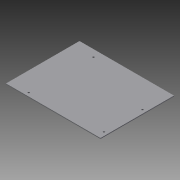
# Autodesk Inventor part: arduino
Saved by Autodesk Inventor 2015 (Build 190159000, 159)
## iProperties
Created: 2014-11-12
Part Number: arduino
Material: Generic
Document SubType Name: Modeling
Designer: Colin
Density: 1 g/cm^3
Appearance: Default
Author: Colin
Autodesk Inventor part; units mm, degrees
ref_plane "YZ Plane" through (0, 0, 0) normal (1, 0, 0) x (0, 1, 0)
ref_plane "XZ Plane" through (0, 0, 0) normal (0, 1, 0) x (-1, 0, 0)
ref_plane "XY Plane" through (0, 0, 0) normal (0, 0, 1) x (1, 0, 0)
sketch "Sketch1" plane through (0, 0, 0) normal (0, 1, 0) x (-1, 0, 0)
  line L0 (0, 0) -> (-68.58, 0)
  line L1 (-68.58, 0) -> (-68.58, -53.34)
  line L2 (-68.58, -53.34) -> (0, -53.34)
  line L3 (0, -53.34) -> (0, 0)
  circle A0 centre (-13.97, -2.54) radius 0.635
  circle A1 centre (-15.24, -48.26) radius 0.635
  circle A2 centre (-66.04, -5.08) radius 0.635
  circle A3 centre (-66.04, -33.02) radius 0.635
  dimension "d0" = 68.58
  dimension "d1" = 53.34
  dimension "d2" = 1.27
  dimension "d3" = 1.27
  dimension "d4" = 13.97
  dimension "d5" = 2.54
  dimension "d6" = 15.24
  dimension "d7" = 5.08
  dimension "d10" = 1.27
  dimension "d11" = 1.27
  dimension "d12" = 50.8
  dimension "d13" = 50.8
  dimension "d14" = 27.94
  dimension "d15" = 15.24
  constraints: 8 end point, 4 centre point, 2 parallel, 1 horizontal, 1 perpendicular
  measures "d0" distance of L0.start L0.end
  measures "d1" distance of L2.end L0.start
  measures "d2" diameter of A0
  measures "d3" diameter of A1
  measures "d4" distance from line of L3 A0.centre
  measures "d5" distance from line of L0 A0.centre
  measures "d6" distance from line of L3 A1.centre
  measures "d7" distance from line of L0 A2.centre
  measures "d10" diameter of A3
  measures "d11" diameter of A2
  measures "d12" horizontal distance of A3.centre A1.centre
  measures "d13" horizontal distance of A1.centre A2.centre
  measures "d14" distance of A2.centre A3.centre
  measures "d15" vertical distance of A1.centre A3.centre
extrude "Extrusion1" add sketch "Sketch1" along normal blind 0.63
body "Solid1"
